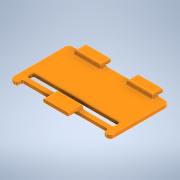
# Autodesk Inventor part: BatteryPlate
Saved by Autodesk Inventor 2021 (Build 250183000, 183)
## iProperties
Created: 2021-05-13
Part Number: BatteryPlate
Material: Generic
Document SubType Name: Modeling
Designer: ermoz
Density: 1 g/cm^3
Appearance: Default
Author: ermoz
Autodesk Inventor part; units mm, degrees
ref_plane "YZ Plane" through (0, 0, 0) normal (1, 0, 0) x (0, 1, 0)
ref_plane "XZ Plane" through (0, 0, 0) normal (0, 1, 0) x (-1, 0, 0)
ref_plane "XY Plane" through (0, 0, 0) normal (0, 0, 1) x (1, 0, 0)
sketch "Sketch1" plane through (0, 0, 0) normal (0, 1, 0) x (-1, 0, 0)
  line L0 (-28.8, -16.8) -> (28.8, -16.8)
  line L1 (28.8, -16.8) -> (28.8, 16.8)
  line L2 (28.8, 16.8) -> (-28.8, 16.8)
  line L3 (-28.8, 16.8) -> (-28.8, -16.8)
  line L4 (-28.8, -16.8) -> (28.8, 16.8) construction
  line L5 (28.8, -16.8) -> (-28.8, 16.8) construction
  point P0 (0, 0)
  dimension "d0" = 33.6
  dimension "d1" = 57.6
  constraints: 12 end point, 2 midpoint, 2 parallel, 1 horizontal, 1 perpendicular
  measures "d0" distance of L0.end L1.end
  measures "d1" distance of L1.end L2.end
extrude "Extrusion1" add sketch "Sketch1" along normal blind 2
fillet "Fillet1" radius 2 4 edges at (28.8, 1, 16.8) (28.8, 1, -16.8) (-28.8, 1, -16.8) (-28.8, 1, 16.8)
sketch "Sketch3" plane through (0, 2, 0) normal (0, 1, 0) x (1, 0, 0)
  line L0 (-22.5, 19.8) -> (-7.5, 19.8)
  line L1 (-7.5, 19.8) -> (-7.5, 13.8)
  line L2 (-7.5, 13.8) -> (-22.5, 13.8)
  line L3 (-22.5, 13.8) -> (-22.5, 19.8)
  line L4 (26.8, 16.8) -> (-26.8, 16.8) projected
  line L5 (-22.5, 19.8) -> (-7.5, 13.8) construction
  line L6 (-7.5, 19.8) -> (-22.5, 13.8) construction
  line L7 (22.5, 19.8) -> (7.5, 19.8)
  line L8 (7.5, 19.8) -> (7.5, 13.8)
  line L9 (7.5, 13.8) -> (22.5, 13.8)
  line L10 (22.5, 13.8) -> (22.5, 19.8)
  line L11 (22.5, 19.8) -> (7.5, 13.8) construction
  line L12 (7.5, 19.8) -> (22.5, 13.8) construction
  line L13 (-7.5, -11.3) -> (7.5, -11.3)
  line L14 (7.5, -11.3) -> (7.5, -19.3)
  line L15 (7.5, -19.3) -> (-7.5, -19.3)
  line L16 (-7.5, -19.3) -> (-7.5, -11.3)
  line L17 (-7.5, -11.3) -> (7.5, -19.3) construction
  line L18 (7.5, -11.3) -> (-7.5, -19.3) construction
  line L19 (25, -7.3) -> (-25, -7.3)
  line L20 (-25, -7.3) -> (-25, -11.3)
  line L21 (-25, -11.3) -> (25, -11.3)
  line L22 (25, -11.3) -> (25, -7.3)
  line L23 (25, -7.3) -> (-25, -11.3) construction
  line L24 (-25, -7.3) -> (25, -11.3) construction
  line L25 (-26.8, -16.8) -> (26.8, -16.8) projected
  line L26 (-25, -13.8) -> (25, -13.8)
  line L27 (25, -13.8) -> (25, -16.8)
  line L28 (25, -16.8) -> (-25, -16.8)
  line L29 (-25, -16.8) -> (-25, -13.8)
  line L30 (-25, -13.8) -> (25, -16.8) construction
  line L31 (25, -13.8) -> (-25, -16.8) construction
  point P0 (0, 0)
  point P1 (-15, 16.8)
  point P2 (15, 16.8)
  point P3 (0, -15.3)
  point P4 (0, -9.3)
  point P5 (0, -9.3)
  point P6 (-7.5, -11.3)
  point P7 (7.5, -11.3)
  point P8 (0, -15.3)
  point P9 (0, -15.3)
  point P10 (0, -15.3)
  dimension "d9" = 15
  dimension "d10" = 6
  dimension "d11" = 15
  dimension "d12" = 15
  dimension "d13" = 6
  dimension "d14" = 15
  dimension "d15" = 15
  dimension "d16" = 8
  dimension "d21" = 4
  dimension "d27" = 2.5
  dimension "d28" = 3
  dimension "d29" = 50
  dimension "d30" = 50
  constraints: 60 end point, 13 midpoint, 10 parallel, 5 horizontal, 5 perpendicular, 3 point on line, 3 vertical alignment, 1 collinear
  measures "d9" distance of L1.end L2.end
  measures "d10" distance of L0.end L1.end
  measures "d11" horizontal distance of point (0, 0) point (-15, 16.8)
  measures "d12" distance of L9.end L8.end
  measures "d13" distance of L7.end L8.end
  measures "d14" horizontal distance of point (0, 0) point (15, 16.8)
  measures "d15" distance of L14.end L15.end
  measures "d16" distance of L13.end L14.end
  measures "d21" distance of L20.end L19.end
  measures "d27" distance between parallel lines of L21 L26
  measures "d28" distance of L28.end L26.start
  measures "d29" distance between parallel lines of L27 L29
  measures "d30" distance of L19.start L19.end
extrude "Extrusion3" add sketch "Sketch3" along normal blind 2 contours L0 L1 L4 L3 | L4 L1 L2 L3 | L10 L9 L8 L4 | L4 L8 L7 L10 | L13 L14 L26 L16 | L26 L14 L25 L16 | L25 L14 L15 L16
extrude "Extrusion4" cut sketch "Sketch3" against normal blind 2 contours L21 L20 L19 L22 L13 | L26 L14 L25 L16 | L16 L25 L29 L26 | L26 L27 L25 L14
fillet "Fillet3" radius 1 16 edges at (15, 2, -13.8) (7.5, 2, -15.3) (22.5, 2, -15.3) (15, 4, -13.8) (7.5, 4, -16.8) (22.5, 4, -16.8) (22.5, 2, -18.3) (7.5, 2, -18.3) (-7.5, 2, -18.3) (-7.5, 4, -16.8) (-22.5, 2, -18.3) (-22.5, 4, -16.8) (-22.5, 2, -15.3) (-15, 2, -13.8) (-15, 4, -13.8) (-7.5, 2, -15.3)
fillet "Fillet4" radius 1 15 edges at (-25, 1, 11.3) (-25, 1, 7.3) (25, 1, 11.3) (25, 1, 7.3) (-7.5, 2, 12.55) (-7.5, 4, 15.3) (7.5, 4, 15.3) (7.5, 2, 12.55) (7.5, 2, 16.55) (-7.5, 2, 16.55) (25, 1, 16.8) (25, 1, 13.8) (-25, 1, 13.8) (-25, 1, 16.8) (0, 2, 13.8)
body "Solid1"
